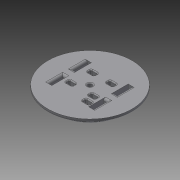
# Autodesk Inventor part: base_toprotate
Saved by Autodesk Inventor 2014 (Build 180170000, 170)
## iProperties
Created: 2014-04-14
Part Number: base_toprotate
Material: Generic
Document SubType Name: Modeling
Designer: t_emanb
Density: 1 g/cm^3
Appearance: Default
Author: t_emanb
Autodesk Inventor part; units mm, degrees
ref_plane "YZ Plane" through (0, 0, 0) normal (1, 0, 0) x (0, 1, 0)
ref_plane "XZ Plane" through (0, 0, 0) normal (0, 1, 0) x (-1, 0, 0)
ref_plane "XY Plane" through (0, 0, 0) normal (0, 0, 1) x (1, 0, 0)
sketch "Sketch1" plane through (0, 0, 0) normal (0, 1, 0) x (-1, 0, 0)
  circle A0 centre (0, 0) radius 53.975
  dimension "d0" = 107.95
  constraints: 1 centre point, 1 coincident
  measures "d0" diameter of A0
extrude "Extrusion1" add sketch "Sketch1" along normal blind 3.81
sketch "Sketch2" plane through (0, 3.81, 0) normal (0, 1, 0) x (1, 0, 0)
  circle A0 centre (0, 0) radius 53.975 projected
  line L0 (0, 53.975) -> (0, -53.975) construction
  line L1 (-23.6474, 6.35) -> (-28.7274, 6.35)
  line L2 (-28.7274, 6.35) -> (-28.7274, 25.4)
  line L3 (-28.7274, 25.4) -> (-23.6474, 25.4)
  line L4 (-23.6474, 25.4) -> (-23.6474, 6.35)
  line L5 (-53.975, 0) -> (53.975, 0) construction
  line L6 (-23.6474, -6.35) -> (-28.7274, -6.35)
  line L7 (-28.7274, -6.35) -> (-28.7274, -25.4)
  line L8 (-28.7274, -25.4) -> (-23.6474, -25.4)
  line L9 (-23.6474, -25.4) -> (-23.6474, -6.35)
  line L10 (23.6474, 6.35) -> (28.7274, 6.35)
  line L11 (28.7274, 6.35) -> (28.7274, 25.4)
  line L12 (28.7274, 25.4) -> (23.6474, 25.4)
  line L13 (23.6474, 25.4) -> (23.6474, 6.35)
  line L14 (23.6474, -6.35) -> (28.7274, -6.35)
  line L15 (28.7274, -6.35) -> (28.7274, -25.4)
  line L16 (23.6474, -25.4) -> (23.6474, -6.35)
  line L17 (28.7274, -25.4) -> (23.6474, -25.4)
  line L18 (-28.7274, 25.4) -> (-23.6474, 25.4)
  line L19 (-23.6474, 6.35) -> (-28.7274, 6.35)
  line L20 (-28.7274, -6.35) -> (-23.6474, -6.35)
  line L21 (-23.6474, -25.4) -> (-28.7274, -25.4)
  line L22 (23.6474, -25.4) -> (28.7274, -25.4)
  line L23 (28.7274, -6.35) -> (23.6474, -6.35)
  line L24 (23.6474, 6.35) -> (28.7274, 6.35)
  line L25 (23.6474, 25.4) -> (28.7274, 25.4)
  dimension "d3" = 5.08
  dimension "d4" = 19.05
  dimension "d6" = 23.6474
  dimension "d10" = 0
  dimension "d11" = 0
  dimension "d12" = 0
  dimension "d13" = 0
  dimension "d14" = 0
  dimension "d15" = 0
  dimension "d16" = 0
  dimension "d17" = 0
  dimension "d76" = 12.7
  constraints: 52 end point, 16 point on line, 12 symmetric about line, 10 perpendicular, 4 point on circle, 3 midpoint, 2 parallel, 1 horizontal, 1 vertical
  measures "d3" distance of L2.end L3.end
  measures "d4" distance of L1.end L2.end
  measures "d6" distance between parallel lines of L0 L4
  measures "d10" distance between parallel lines of L3 L18
  measures "d11" distance between parallel lines of L1 L19
  measures "d12" distance between parallel lines of L6 L20
  measures "d13" distance between parallel lines of L8 L21
  measures "d14" distance between parallel lines of L17 L22
  measures "d15" distance between parallel lines of L14 L23
  measures "d16" distance between parallel lines of L10 L24
  measures "d17" distance between parallel lines of L12 L25
  measures "d76" distance between parallel lines of L20 L19
extrude "Extrusion3" cut sketch "Sketch2" against normal through all contours L1 L2 L3 L4 | L9 L8 L7 L6 | L13 L12 L11 L10 | L14 L15 L17 L16
sketch "Sketch5" plane through (0, 0, 0) normal (0, -1, 0) x (1, 0, 0)
  line L0 (28.7274, 25.4) -> (28.7274, 6.35) projected
  line L1 (28.7274, 6.35) -> (23.6474, 6.35) projected
  line L2 (23.6474, 6.35) -> (23.6474, 25.4) projected
  line L3 (23.6474, 25.4) -> (28.7274, 25.4) projected
  line L4 (-28.7274, -6.35) -> (-23.6474, -6.35) projected
  line L5 (-23.6474, -6.35) -> (-23.6474, -25.4) projected
  line L6 (-23.6474, -25.4) -> (-28.7274, -25.4) projected
  line L7 (-28.7274, -25.4) -> (-28.7274, -6.35) projected
  line L8 (-28.7274, 25.4) -> (-23.6474, 25.4) projected
  line L9 (-23.6474, 25.4) -> (-23.6474, 6.35) projected
  line L10 (-23.6474, 6.35) -> (-28.7274, 6.35) projected
  line L11 (-28.7274, 6.35) -> (-28.7274, 25.4) projected
  line L12 (28.7274, -6.35) -> (28.7274, -25.4) projected
  line L13 (28.7274, -25.4) -> (23.6474, -25.4) projected
  line L14 (23.6474, -25.4) -> (23.6474, -6.35) projected
  line L15 (23.6474, -6.35) -> (28.7274, -6.35) projected
  arc A0 (-53.975, 0) -> (-53.975, 0) centre (0, 0) ccw projected
  circle A1 centre (0, 0) radius 43.815
  dimension "d30" = 87.63
  constraints: 1 centre point, 1 coincident
  measures "d30" diameter of A1
extrude "Extrusion6" add sketch "Sketch5" along normal blind 7.874 contours A1
sketch "Sketch6" plane through (0, -7.874, 0) normal (0, -1, 0) x (1, 0, 0)
  line L0 (28.7274, 25.4) -> (28.7274, 6.35) projected
  circle A0 centre (0, 0) radius 43.815 projected
  line L1 (0, 0) -> (43.815, 0) construction
  line L2 (-9.525, 36.83) -> (9.525, 36.83)
  line L3 (9.525, 36.83) -> (9.525, 30.48)
  line L4 (9.525, 30.48) -> (-9.525, 30.48)
  line L5 (-9.525, 30.48) -> (-9.525, 36.83)
  line L6 (0, 0) -> (0, 43.815) construction
  line L7 (-9.525, -36.83) -> (9.525, -36.83)
  line L8 (9.525, -36.83) -> (9.525, -30.48)
  line L9 (9.525, -30.48) -> (-9.525, -30.48)
  line L10 (-9.525, -30.48) -> (-9.525, -36.83)
  dimension "d33" = 6.35
  dimension "d34" = 19.05
  dimension "d35" = 30.48
  constraints: 20 end point, 4 symmetric about line, 3 parallel, 2 perpendicular, 2 point on circle, 1 horizontal, 1 other
  measures "d33" distance of L4.end L2.start
  measures "d34" distance of L2.start L2.end
  measures "d35" distance between parallel lines of L1 L4
extrude "Extrusion7" cut sketch "Sketch6" against normal blind 8.89 contours L2 L3 L4 L5 | L10 L9 L8 L7
sketch "Sketch7" plane through (0, 3.81, 0) normal (0, 1, 0) x (1, 0, 0)
  arc A0 (-53.975, 0) -> (-53.975, 0) centre (0, 0) ccw projected
  circle A1 centre (0, 0) radius 1.4224
  dimension "d38" = 2.8448
  constraints: 1 centre point, 1 coincident
  measures "d38" diameter of A1
extrude "Extrusion8" cut sketch "Sketch7" against normal through all contours A1
sketch "Sketch8" plane through (0, 3.81, 0) normal (0, 1, 0) x (1, 0, 0)
  circle A0 centre (0, 0) radius 1.4224 projected
  arc A1 (-53.975, 0) -> (-53.975, 0) centre (0, 0) ccw projected
  circle A2 centre (0, 0) radius 2.921
  dimension "d41" = 5.842
  constraints: 1 centre point, 1 coincident
  measures "d41" diameter of A2
extrude "Extrusion9" cut sketch "Sketch8" against normal blind 9.144 contours A2
sketch "Sketch9" plane through (0, -7.874, 0) normal (0, -1, 0) x (1, 0, 0)
  circle A0 centre (0, 0) radius 1.4224 projected
  line L0 (9.525, -36.83) -> (-9.525, -36.83) projected
  circle A1 centre (0, 0) radius 43.815 projected
  line L1 (-16.383, -12.7) -> (-7.747, -12.7)
  line L2 (-7.747, -12.7) -> (-7.747, -17.78)
  line L3 (-7.747, -17.78) -> (-16.383, -17.78)
  line L4 (-16.383, -17.78) -> (-16.383, -12.7)
  line L5 (0, 0) -> (0, -36.83) construction
  line L6 (16.383, -12.7) -> (7.747, -12.7)
  line L7 (7.747, -12.7) -> (7.747, -17.78)
  line L8 (7.747, -17.78) -> (16.383, -17.78)
  line L9 (16.383, -17.78) -> (16.383, -12.7)
  line L10 (-10.16, -12.7) -> (-10.16, -17.78) construction
  line L11 (-12.065, -12.7) -> (-12.065, -17.78) construction
  line L12 (-18.796, 12.7) -> (-10.16, 12.7)
  line L13 (-10.16, 12.7) -> (-10.16, 7.62)
  line L14 (-10.16, 7.62) -> (-18.796, 7.62)
  line L15 (-18.796, 7.62) -> (-18.796, 12.7)
  line L16 (18.796, 12.7) -> (10.16, 12.7)
  line L17 (10.16, 12.7) -> (10.16, 7.62)
  line L18 (10.16, 7.62) -> (18.796, 7.62)
  line L19 (18.796, 7.62) -> (18.796, 12.7)
  line L20 (12.7, 17.78) -> (21.336, 17.78)
  line L21 (21.336, 17.78) -> (21.336, 22.86)
  line L22 (21.336, 22.86) -> (12.7, 22.86)
  line L23 (12.7, 22.86) -> (12.7, 17.78)
  dimension "d44" = 5.08
  dimension "d45" = 8.636
  dimension "d46" = 12.7
  dimension "d67" = 1.905
  dimension "d68" = 10.16
  dimension "d69" = 7.62
  dimension "d70" = 10.16
  dimension "d71" = 8.636
  dimension "d72" = 5.08
  dimension "d77" = 8.636
  dimension "d78" = 5.08
  dimension "d79" = 12.7
  dimension "d80" = 17.78
  constraints: 46 end point, 8 symmetric about line, 6 parallel, 4 perpendicular, 3 horizontal, 3 midpoint, 2 point on line
  measures "d44" distance of L1.end L2.end
  measures "d45" distance of L2.end L3.end
  measures "d46" distance from line of A0.centre L1
  measures "d67" distance between parallel lines of L11 L10
  measures "d68" distance between parallel lines of L5 L10
  measures "d69" distance from line of A0.centre L14
  measures "d70" distance from line of A0.centre L13
  measures "d71" distance of L13.end L14.end
  measures "d72" distance of L14.end L12.start
  measures "d77" distance of L20.start L20.end
  measures "d78" distance of L22.end L20.start
  measures "d79" distance between parallel lines of L5 L23
  measures "d80" distance from line of A0.centre L20
extrude "Extrusion10" cut sketch "Sketch9" against normal through all contours L1 L2 L3 L4 | L9 L8 L7 L6 | L12 L13 L14 L15 | L19 L18 L17 L16 | L23 L22 L21 L20
sketch "Sketch10" plane through (0, 0, 0) normal (1, 0, 0) x (0, 1, 0)
  line L0 (3.81, -53.975) -> (3.81, 53.975) projected
  line L1 (0, 53.975) -> (0, -53.975) projected
  line L2 (-7.874, 43.815) -> (-7.874, -43.815) projected
  line L3 (0, -43.815) -> (0, 43.815) projected
  arc A0 (0, -45.5253) -> (0, -52.2647) centre (1.778, -48.895) ccw
  line L4 (0, -53.975) -> (3.81, -53.975)
  line L5 (-2.032, -48.895) -> (0, -48.895)
  line L6 (-2.032, -48.895) -> (-2.032, -43.815) construction
  point P0 (0, 0)
  dimension "d50" = 7.62
  dimension "d51" = 5.08
  dimension "d53" = 1.778
  dimension "d58" = 5.842
  constraints: 6 end point, 3 perpendicular, 3 point on circle, 3 point on line, 1 centre point, 1 tangent
  measures "d50" diameter of A0
  measures "d51" distance from line of L4 A0.centre
  measures "d53" distance from line of L1 A0.centre
  measures "d58" distance between parallel lines of L0 L6
revolve "Revolution2" add sketch "Sketch10" angle 360 about axis through (0, -2.032, -48.895) along (0, 1, 0) picked at (-0.228, -46.8025) contours L1 L5 A0
pattern_circular "Circular Pattern1" count 12 over 360 about axis through (0, -10, 0) along (0, 1, 0) of "Revolution2"
fillet "Fillet1" radius 1.27 8 edges at (-9.525, -7.874, 33.655) (0, -7.874, 36.83) (9.525, -7.874, 33.655) (0, -7.874, 30.48) (0, -7.874, -30.48) (9.525, -7.874, -33.655) (0, -7.874, -36.83) (-9.525, -7.874, -33.655)
fillet "Fillet2" radius 2.286 4 edges at (9.525, 1.016, 33.655) (-9.525, 1.016, 33.655) (9.525, 1.016, -33.655) (-9.525, 1.016, -33.655)
fillet "Fillet4" radius 2.794 8 edges at (26.1874, 3.81, -6.35) (26.1874, 3.81, 6.35) (-26.1874, 3.81, 6.35) (-26.1874, 3.81, -6.35) (-28.7274, 3.81, 15.875) (-28.7274, 3.81, -15.875) (28.7274, 3.81, 15.875) (28.7274, 3.81, -15.875)
sketch "Sketch11" plane through (0, -7.874, 0) normal (0, -1, 0) x (1, 0, 0)
  circle A0 centre (0, 0) radius 1.4224 projected
  circle A1 centre (0, 0) radius 43.815 projected
  circle A2 centre (0, 0) radius 4.5085
  dimension "d63" = 9.017
  constraints: 1 centre point, 1 coincident
  measures "d63" diameter of A2
extrude "Extrusion11" cut sketch "Sketch11" against normal blind 0.508 contours A2
fillet "Fillet5" radius 1.27 40 edges at (-16.383, -7.874, -15.24) (-12.065, -7.874, -12.7) (-7.747, -7.874, -15.24) (-12.065, -7.874, -17.78) (12.065, -7.874, -17.78) (7.747, -7.874, -15.24) (12.065, -7.874, -12.7) (16.383, -7.874, -15.24) (16.383, -2.032, -17.78) (7.747, -2.032, -17.78) (7.747, -2.032, -12.7) (16.383, -2.032, -12.7) (-7.747, -2.032, -12.7) (-16.383, -2.032, -17.78) (-16.383, -2.032, -12.7) (-7.747, -2.032, -17.78) (18.796, -7.874, 10.16) (14.478, -7.874, 7.62) (10.16, -7.874, 10.16) (14.478, -7.874, 12.7) (-18.796, -7.874, 10.16) (-14.478, -7.874, 12.7) (-10.16, -7.874, 10.16) (-14.478, -7.874, 7.62) (10.16, -2.032, 7.62) (10.16, -2.032, 12.7) (-18.796, -2.032, 12.7) (18.796, -2.032, 7.62) (-10.16, -2.032, 7.62) (-18.796, -2.032, 7.62) (-10.16, -2.032, 12.7) (18.796, -2.032, 12.7) (21.336, -7.874, 20.32) (17.018, -7.874, 17.78) (12.7, -7.874, 20.32) (17.018, -7.874, 22.86) (12.7, -2.032, 17.78) (12.7, -2.032, 22.86) (21.336, -2.032, 22.86) (21.336, -2.032, 17.78)
fillet "Fillet6" radius 1.27 42 edges at (-12.065, 3.81, -12.7) (-16.011, 3.81, -13.072) (-16.383, 3.81, -15.24) (-16.011, 3.81, -17.408) (-12.065, 3.81, -17.78) (-8.119, 3.81, -17.408) (-7.747, 3.81, -15.24) (-8.119, 3.81, -13.072) (-14.478, 3.81, 12.7) (-18.424, 3.81, 12.328) (-18.796, 3.81, 10.16) (-18.424, 3.81, 7.992) (-14.478, 3.81, 7.62) (-10.532, 3.81, 7.992) (-10.16, 3.81, 10.16) (-10.532, 3.81, 12.328) (-2.921, 3.81, 0) (12.065, 3.81, -17.78) (16.011, 3.81, -17.408) (16.383, 3.81, -15.24) (16.011, 3.81, -13.072) (12.065, 3.81, -12.7) (8.119, 3.81, -13.072) (7.747, 3.81, -15.24) (8.119, 3.81, -17.408) (14.478, 3.81, 12.7) (10.532, 3.81, 12.328) (10.16, 3.81, 10.16) (10.532, 3.81, 7.992) (14.478, 3.81, 7.62) (18.424, 3.81, 7.992) (18.796, 3.81, 10.16) (18.424, 3.81, 12.328) (-1.4224, -7.366, 0) (21.336, 3.81, 20.32) (20.964, 3.81, 22.488) (17.018, 3.81, 22.86) (13.072, 3.81, 22.488) (12.7, 3.81, 20.32) (13.072, 3.81, 18.152) (17.018, 3.81, 17.78) (20.964, 3.81, 18.152)
fillet "Fillet7" radius 1.27 3 edges at (-43.815, 0, 0) (53.975, 0, 0) (-43.815, -7.874, 0)
fillet "Fillet8" radius 0.508 2 edges at (-2.921, -5.334, 0) (-1.4224, -5.334, 0)
body "Solid1"
